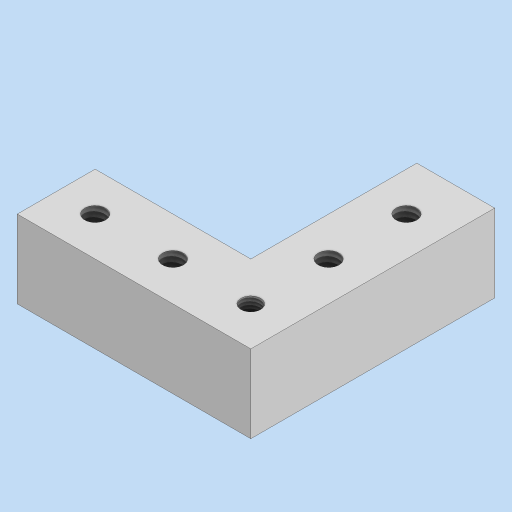
# Autodesk Inventor part: STRU_004_DoubleBillet_90_2.25in
Saved by Autodesk Inventor 2024.3 (Build 283343000, 343)
## iProperties
Created: 2024-07-23
Part Number: STRU_004_DoubleBillet_90_2.25in
Material: Generic
Document SubType Name: Modeling
Designer: bryan
Density: 1 g/cm^3
Appearance: Default
Author: bryan
Autodesk Inventor part; units mm, degrees
ref_plane "YZ Plane" through (0, 0, 0) normal (1, 0, 0) x (0, 1, 0)
ref_plane "XZ Plane" through (0, 0, 0) normal (0, 1, 0) x (-1, 0, 0)
ref_plane "XY Plane" through (0, 0, 0) normal (0, 0, 1) x (1, 0, 0)
sketch "Sketch1" plane through (0, 0, 0) normal (0, 1, 0) x (-1, 0, 0)
  line L0 (0, 0) -> (57.15, 0)
  line L1 (57.15, 0) -> (57.15, -19.05)
  line L2 (57.15, -19.05) -> (19.05, -19.05)
  line L3 (19.05, -19.05) -> (19.05, -59.69)
  line L4 (19.05, -59.69) -> (0, -59.69)
  line L5 (0, -59.69) -> (0, 0)
  circle A0 centre (28.575, -9.525) radius 2.5527
  circle A1 centre (47.625, -9.525) radius 2.5527
  line L6 (19.05, -19.05) -> (0, 0) construction
  circle A2 centre (9.525, -28.575) radius 2.5527
  circle A3 centre (9.525, -47.625) radius 2.5527
  circle A4 centre (9.525, -9.525) radius 2.413
  point P0 (57.15, -9.525)
  dimension "d0" = 19.05
  dimension "d1" = 19.05
  dimension "d2" = 59.69
  dimension "d3" = 57.15
  dimension "d4" = 5.1054
  dimension "d5" = 28.575
  dimension "d6" = 19.05
  dimension "d19" = 4.826
  constraints: 14 end point, 5 centre point, 5 perpendicular, 2 horizontal alignment, 2 midpoint, 2 symmetric about line, 1 equal radius, 1 horizontal, 2 other
  measures "d0" distance of L0.end L1.end
  measures "d1" distance of L3.end L4.end
  measures "d2" distance between parallel lines of L4 L0
  measures "d3" distance of L0.start L0.end
  measures "d4" diameter of A1
  measures "d5" distance from line of L5 A0.centre
  measures "d6" distance of A0.centre A1.centre
  measures "d19" diameter of A4
extrude "Extrusion1" add sketch "Sketch1" along normal mid plane 19.05
thread "Thread1" size "1/4-20 UNC" class "2B" standard "ANSI Unified Screw Threads" full length
thread "Thread2" size "1/4-20 UNC" class "2B" standard "ANSI Unified Screw Threads" full length
thread "Thread3" size "1/4-20 UNC" class "2B" standard "ANSI Unified Screw Threads" full length
thread "Thread4" size "1/4-20 UNC" class "2B" standard "ANSI Unified Screw Threads" full length
thread "Thread5" size "10-32 UNF" class "2B" standard "ANSI Unified Screw Threads" full length
body "Solid1"
